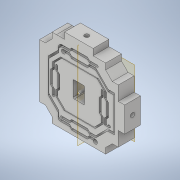
# Autodesk Inventor part: 20_Cube_Inser_Flexuremanipulator_m3_lc_fibermount_v3
Saved by Autodesk Inventor 2022 (Build 260153000, 153)
## iProperties
Created: 2021-03-01
Part Number: 20_Cube_Inser_Flexuremanipulator_m3_lc_fibermount_v3
Material: Generic
Document SubType Name: Modeling
Designer: diederichbenedict
Density: 1 g/cm^3
Appearance: Default
Author: diederichbenedict
Autodesk Inventor part; units mm, degrees
ref_plane "YZ Plane" through (0, 0, 0) normal (1, 0, 0) x (0, 1, 0)
ref_plane "XZ Plane" through (0, 0, 0) normal (0, 1, 0) x (-1, 0, 0)
ref_plane "XY Plane" through (0, 0, 0) normal (0, 0, 1) x (1, 0, 0)
ref_plane "Work Plane1" through (7.88, 34.1, 0) normal (0, 0, 1) x (-1, 0, 0)
sketch "Sketch1" plane through (7.88, 34.1, 0) normal (0, 0, 1) x (-1, 0, 0)
  circle A0 centre (24.85, 16.97) radius 1.6106 projected
  line L0 (10.689, 37.795) -> (10.689, 41.96) projected
  line L1 (10.689, 37.795) -> (10.689, 34.7795) projected
  line L2 (10.689, 34.7795) -> (7.0405, 31.131) projected
  line L3 (7.0405, 31.131) -> (4.025, 31.131) projected
  line L4 (4.025, 31.131) -> (-0.14, 31.131) projected
  line L5 (-0.14, 31.131) -> (-0.14, 2.809) projected
  line L6 (-0.14, 2.809) -> (4.025, 2.809) projected
  line L7 (4.025, 2.809) -> (7.0405, 2.809) projected
  line L8 (7.0405, 2.809) -> (10.689, -0.8395) projected
  line L9 (10.689, -0.8395) -> (10.689, -3.855) projected
  line L10 (10.689, -3.855) -> (10.689, -8.02) projected
  line L11 (10.689, -8.02) -> (39.011, -8.02) projected
  line L12 (39.011, -8.02) -> (39.011, -3.855) projected
  line L13 (39.011, -3.855) -> (39.011, -0.8395) projected
  line L14 (39.011, -0.8395) -> (42.6595, 2.809) projected
  line L15 (42.6595, 2.809) -> (45.675, 2.809) projected
  line L16 (45.675, 2.809) -> (45.675, 31.131) projected
  line L17 (42.6595, 31.131) -> (45.675, 31.131) projected
  line L18 (42.6595, 31.131) -> (39.011, 34.7795) projected
  line L19 (39.011, 34.7795) -> (39.011, 37.795) projected
  line L20 (39.011, 41.96) -> (39.011, 37.795) projected
  line L21 (10.689, 41.96) -> (39.011, 41.96) projected
  line L22 (30.605, 38.2115) -> (36.5749, 38.2115) projected
  arc A1 (37.9461, 36.6239) -> (36.5749, 38.2115) centre (36.5749, 36.8256) ccw projected
  line L23 (37.9461, 36.6239) -> (37.9461, 33.9428) projected
  line L24 (44.1756, 27.7133) -> (37.9461, 33.9428) projected
  line L25 (44.1756, 6.1367) -> (44.1756, 27.7133) projected
  line L26 (37.9461, -0.0928) -> (44.1756, 6.1367) projected
  line L27 (37.9461, -0.0928) -> (37.9461, -1.4371) projected
  arc A2 (36.0225, -4.2715) -> (37.9461, -1.4371) centre (34.8961, -1.4371) ccw projected
  line L28 (36.0225, -4.2715) -> (30.605, -4.2715) projected
  line L29 (29.3555, -5.521) -> (30.605, -4.2715) projected
  line L30 (19.3595, -5.521) -> (29.3555, -5.521) projected
  line L31 (18.11, -4.2715) -> (19.3595, -5.521) projected
  line L32 (13.2194, -4.2715) -> (18.11, -4.2715) projected
  arc A3 (13.2194, -3.022) -> (13.2194, -4.2715) centre (13.2194, -3.6467) ccw projected
  line L33 (18.11, -3.022) -> (13.2194, -3.022) projected
  line L34 (19.3595, -4.2715) -> (18.11, -3.022) projected
  line L35 (29.3555, -4.2715) -> (19.3595, -4.2715) projected
  line L36 (30.605, -3.022) -> (29.3555, -4.2715) projected
  line L37 (30.605, -3.022) -> (34.8506, -3.022) projected
  arc A4 (34.8506, -3.022) -> (37.5296, -0.9944) centre (34.8506, -0.2385) ccw projected
  line L38 (37.5296, -0.9944) -> (37.5296, 1.1567) projected
  line L39 (43.7591, 7.3862) -> (37.5296, 1.1567) projected
  line L40 (43.7591, 26.4638) -> (43.7591, 7.3862) projected
  line L41 (37.5296, 32.6933) -> (43.7591, 26.4638) projected
  line L42 (37.5296, 35.8344) -> (37.5296, 32.6933) projected
  arc A5 (37.5296, 35.8344) -> (36.402, 36.962) centre (36.402, 35.8344) ccw projected
  line L43 (30.605, 36.962) -> (36.402, 36.962) projected
  line L44 (29.3555, 38.2115) -> (30.605, 36.962) projected
  line L45 (19.3595, 38.2115) -> (29.3555, 38.2115) projected
  line L46 (18.11, 36.962) -> (19.3595, 38.2115) projected
  line L47 (14.4288, 36.962) -> (18.11, 36.962) projected
  arc A6 (15.7715, 38.3046) -> (14.4288, 36.962) centre (14.4288, 38.3046) ccw projected
  line L48 (15.7715, 38.2115) -> (15.7715, 38.3046) projected
  line L49 (18.11, 38.2115) -> (15.7715, 38.2115) projected
  line L50 (19.3595, 39.461) -> (18.11, 38.2115) projected
  line L51 (29.3555, 39.461) -> (19.3595, 39.461) projected
  line L52 (30.605, 38.2115) -> (29.3555, 39.461) projected
  line L53 (6.524, 28.5756) -> (14.0774, 36.129) projected
  line L54 (14.0774, 36.129) -> (18.11, 36.129) projected
  line L55 (18.11, 36.129) -> (19.3595, 34.8795) projected
  line L56 (19.3595, 34.8795) -> (29.3555, 34.8795) projected
  line L57 (29.3555, 34.8795) -> (30.605, 36.129) projected
  line L58 (30.605, 36.129) -> (35.7862, 36.129) projected
  arc A7 (35.7862, 34.8795) -> (35.7862, 36.129) centre (35.7862, 35.5043) ccw projected
  line L59 (35.7862, 34.8795) -> (30.605, 34.8795) projected
  line L60 (30.605, 34.8795) -> (29.3555, 33.63) projected
  line L61 (29.3555, 33.63) -> (19.3595, 33.63) projected
  line L62 (19.3595, 33.63) -> (18.11, 34.8795) projected
  line L63 (18.11, 34.8795) -> (14.0774, 34.8795) projected
  line L64 (14.0774, 34.8795) -> (6.524, 27.3261) projected
  line L65 (6.524, 27.3261) -> (2.7755, 27.3261) projected
  line L66 (2.7755, 27.3261) -> (2.7755, 6.9149) projected
  line L67 (2.7755, 6.9149) -> (6.223, 6.9149) projected
  line L68 (6.223, 6.9149) -> (14.0774, -0.9395) projected
  line L69 (14.0774, -0.9395) -> (18.11, -0.9395) projected
  line L70 (18.11, -0.9395) -> (19.3595, 0.31) projected
  line L71 (19.3595, 0.31) -> (29.3555, 0.31) projected
  line L72 (29.3555, 0.31) -> (30.605, -0.9395) projected
  line L73 (30.605, -0.9395) -> (33.3749, -0.9395) projected
  arc A8 (34.6244, -2.189) -> (33.3749, -0.9395) centre (34.6244, -0.9395) ccw projected
  line L74 (34.6244, -2.189) -> (30.605, -2.189) projected
  line L75 (30.605, -2.189) -> (29.3555, -0.9395) projected
  line L76 (29.3555, -0.9395) -> (19.3595, -0.9395) projected
  line L77 (19.3595, -0.9395) -> (18.11, -2.189) projected
  line L78 (18.11, -2.189) -> (14.0774, -2.189) projected
  line L79 (14.0774, -2.189) -> (6.223, 5.6654) projected
  line L80 (2.359, 5.6654) -> (6.223, 5.6654) projected
  line L81 (2.359, 28.5756) -> (2.359, 5.6654) projected
  line L82 (6.524, 28.5756) -> (2.359, 28.5756) projected
  line L83 (7.357, 21.135) -> (7.357, 12.805) projected
  line L84 (8.6065, 11.5555) -> (7.357, 12.805) projected
  line L85 (8.6065, 9.1359) -> (8.6065, 11.5555) projected
  line L86 (8.6065, 7.7897) -> (8.6065, 9.1359) projected
  line L87 (13.1707, 3.2255) -> (8.6065, 7.7897) projected
  line L88 (35.5512, 3.2255) -> (13.1707, 3.2255) projected
  line L89 (40.2764, 7.9507) -> (35.5512, 3.2255) projected
  line L90 (40.2764, 11.5555) -> (40.2764, 7.9507) projected
  line L91 (41.5259, 12.805) -> (40.2764, 11.5555) projected
  line L92 (41.5259, 21.135) -> (41.5259, 12.805) projected
  line L93 (40.2764, 22.3845) -> (41.5259, 21.135) projected
  line L94 (40.2764, 26.4297) -> (40.2764, 22.3845) projected
  arc A9 (41.5259, 26.4297) -> (40.2764, 26.4297) centre (40.9011, 26.4297) ccw projected
  line L95 (41.5259, 22.3845) -> (41.5259, 26.4297) projected
  line L96 (42.7754, 21.135) -> (41.5259, 22.3845) projected
  line L97 (42.7754, 12.805) -> (42.7754, 21.135) projected
  line L98 (41.5259, 11.5555) -> (42.7754, 12.805) projected
  line L99 (41.5259, 8.0241) -> (41.5259, 11.5555) projected
  line L100 (36.3107, 2.809) -> (41.5259, 8.0241) projected
  line L101 (12.3377, 2.809) -> (36.3107, 2.809) projected
  line L102 (7.357, 7.7897) -> (12.3377, 2.809) projected
  line L103 (7.357, 9.1113) -> (7.357, 7.7897) projected
  line L104 (7.357, 11.5555) -> (7.357, 9.1113) projected
  line L105 (6.1075, 12.805) -> (7.357, 11.5555) projected
  line L106 (6.1075, 21.135) -> (6.1075, 12.805) projected
  line L107 (7.357, 22.3845) -> (6.1075, 21.135) projected
  line L108 (7.357, 25.5514) -> (7.357, 22.3845) projected
  line L109 (6.3945, 25.5514) -> (7.357, 25.5514) projected
  arc A10 (5.61, 26.3074) -> (6.3945, 25.5514) centre (5.61, 25.5223) ccw projected
  line L110 (8.6065, 26.3074) -> (5.61, 26.3074) projected
  line L111 (8.6065, 22.3845) -> (8.6065, 26.3074) projected
  line L112 (7.357, 21.135) -> (8.6065, 22.3845) projected
  line L113 (9.4395, 8.2659) -> (9.4395, 11.5555) projected
  line L114 (9.4395, 11.5555) -> (10.689, 12.805) projected
  line L115 (10.689, 12.805) -> (10.689, 21.135) projected
  line L116 (10.689, 21.135) -> (9.4395, 22.3845) projected
  line L117 (9.4395, 22.3845) -> (9.4395, 26.2659) projected
  line L118 (9.4395, 26.2659) -> (14.3046, 31.131) projected
  line L119 (14.3046, 31.131) -> (34.1168, 31.131) projected
  line L120 (34.1168, 31.131) -> (39.4434, 25.8045) projected
  line L121 (39.4434, 25.8045) -> (39.4434, 22.3845) projected
  line L122 (39.4434, 22.3845) -> (38.1939, 21.135) projected
  line L123 (38.1939, 21.135) -> (38.1939, 12.805) projected
  line L124 (38.1939, 12.805) -> (39.4434, 11.5555) projected
  line L125 (39.4434, 11.5555) -> (39.4434, 8.8128) projected
  arc A11 (38.1939, 8.8128) -> (39.4434, 8.8128) centre (38.8186, 8.8128) ccw projected
  line L126 (38.1939, 8.8128) -> (38.1939, 11.5555) projected
  line L127 (38.1939, 11.5555) -> (36.9444, 12.805) projected
  line L128 (36.9444, 12.805) -> (36.9444, 21.135) projected
  line L129 (36.9444, 21.135) -> (38.1939, 22.3845) projected
  line L130 (38.1939, 22.3845) -> (38.1939, 25.8045) projected
  line L131 (38.1939, 25.8045) -> (33.2838, 30.7145) projected
  line L132 (33.2838, 30.7145) -> (15.1376, 30.7145) projected
  line L133 (15.1376, 30.7145) -> (10.689, 26.2659) projected
  line L134 (10.689, 26.2659) -> (10.689, 22.3845) projected
  line L135 (10.689, 22.3845) -> (11.9385, 21.135) projected
  line L136 (11.9385, 21.135) -> (11.9385, 12.805) projected
  line L137 (11.9385, 12.805) -> (10.689, 11.5555) projected
  line L138 (10.689, 11.5555) -> (10.689, 8.2659) projected
  arc A12 (9.4395, 8.2659) -> (10.689, 8.2659) centre (10.0643, 8.2659) ccw projected
  line L139 (7.88, -4.18) -> (3.7, 0) construction
  line L140 (7.88, 38.28) -> (3.7, 34.1) projected
  line L141 (46, 34.1) -> (41.82, 38.28) construction
  line L142 (46, 0) -> (41.82, -4.18) construction
  line L143 (41.82, -8) -> (41.82, -4.18) construction
  line L144 (46, 0) -> (49.7, 0) construction
  line L145 (46, 34.1) -> (49.7, 34.1) construction
  line L146 (41.82, 42.1) -> (41.82, 38.28) construction
  line L147 (7.88, 42.1) -> (7.88, 38.28) construction
  line L148 (0, 34.1) -> (4.1, 34.1) construction
  line L149 (3.7, 0) -> (0, 0) construction
  line L150 (7.88, -8) -> (7.88, -4.18) construction
  line L151 (39.011, -8.02) -> (41.82, -8)
  line L152 (41.82, -8) -> (41.793, -4.207)
  line L153 (46, 0) -> (41.793, -4.207)
  line L154 (10.689, -8.02) -> (7.88, -8.02)
  line L155 (7.88, -8.02) -> (7.88, -4.207)
  line L156 (7.88, -4.207) -> (3.7, 0)
  line L157 (3.7, 0) -> (0, 0)
  line L158 (0, 0) -> (-0.14, 0)
  line L159 (-0.14, 0) -> (-0.14, 2.809)
  line L160 (-0.14, 31.131) -> (-0.14, 34.1)
  line L161 (-0.14, 34.1) -> (3.7, 34.1)
  line L162 (7.88, 38.28) -> (7.88, 41.96)
  line L163 (7.88, 38.28) -> (11.56, 38.28) construction
  line L164 (7.88, 41.96) -> (10.689, 41.96)
  line L165 (39.011, 41.96) -> (41.82, 41.96)
  line L166 (41.82, 41.96) -> (41.82, 38.28)
  line L167 (46, 34.1) -> (41.82, 38.28)
  line L168 (46, 34.1) -> (49.7, 34.1)
  line L169 (49.7, 34.1) -> (49.7, 0)
  line L170 (49.7, 0) -> (46, 0)
  point P0 (7.88, 34.1)
  dimension "d0" = 0
  dimension "d1" = 90
  constraints: 40 end point, 7 perpendicular, 6 point on line, 3 collinear, 1 horizontal, 1 vertical
  measures "d0" distance from line of L154.end L150
  measures "d1" angle of L163 L162
extrude "Extrusion1" add sketch "Sketch1" along normal blind 10
sketch "Sketch3" plane through (8.02, 0, 0) normal (1, 0, 0) x (0, 0, -1)
  line L0 (0, 0) -> (0, 34.1) projected
  line L1 (0, 34.1) -> (-10, 34.1) projected
  line L2 (-10, 0) -> (-10, 34.1) projected
  line L3 (0, 0) -> (-10, 0) projected
  line L4 (0, 21.295) -> (0, 12.965) projected
  line L5 (0, 21.295) -> (-10, 21.295) projected
  line L6 (-10, 12.965) -> (-10, 21.295) projected
  line L7 (0, 12.965) -> (-10, 12.965) projected
  point P0 (0, 0)
  point P1 (-5, 17.13)
hole "Hole1" at (8.02, 17.13, 5) direction (-1, 0, 0) diameter 4.9 depth 12.0785
sketch "Sketch6" plane through (5.1045, 6.7739, 0) normal (1, 0, 0) x (0, 0, -1)
  line L0 (0, 14.5211) -> (0, 6.1911) projected
  line L1 (0, 14.5211) -> (-10, 14.5211) projected
  line L2 (-10, 6.1911) -> (-10, 14.5211) projected
  line L3 (0, 6.1911) -> (-10, 6.1911) projected
  circle A0 centre (-5, 10.3561) radius 2.45 projected
  line L4 (-5, 8.8561) -> (-5, 11.8561) construction
  line L5 (-2.2, 8.8561) -> (-2.2, 11.8561)
  line L6 (-7.8, 11.8561) -> (-7.8, 8.8561)
  arc A1 (-7.8, 8.8561) -> (-2.2, 8.8561) centre (-5, 8.8561) ccw
  arc A2 (-2.2, 11.8561) -> (-7.8, 11.8561) centre (-5, 11.8561) ccw
  line L7 (-5, 10.3561) -> (-2, 10.3561) construction
  point P0 (0, -6.7739)
  dimension "d21" = 1.5
  dimension "d22" = 90
  dimension "d23" = 5.6
  constraints: 10 end point, 4 point on circle, 4 tangent, 2 centre point, 1 horizontal, 1 midpoint, 1 parallel, 1 perpendicular, 1 vertical
  measures "d21" distance of L7.start L4.end
  measures "d22" angle of L7 L4
  measures "d23" diameter of A2
extrude "Extrusion4" cut sketch "Sketch6" against normal up to surface (7.9135 mm away) contours A2 L5 A1 L3 L6 L1 | L1 A2 | A1 L3 | A0
pattern_circular "Circular Pattern3" count 2 over 90 about axis through (-16.97, 17.13, 0) along (0, 0, 1) of "Hole1", "Extrusion4"
sketch "Sketch7" plane through (7.88, 34.1, 10) normal (0, 0, 1) x (1, 0, 0)
  arc A0 (-37.9461, -36.6239) -> (-36.5749, -38.2115) centre (-36.5749, -36.8256) ccw projected
  line L0 (-37.9461, -36.6239) -> (-37.9461, -33.9428) projected
  line L1 (-37.9461, -33.9428) -> (-44.1756, -27.7133) projected
  line L2 (-44.1756, -27.7133) -> (-44.1756, -6.1367) projected
  line L3 (-44.1756, -6.1367) -> (-37.9461, 0.0928) projected
  line L4 (-37.9461, 0.0928) -> (-37.9461, 1.4371) projected
  arc A1 (-36.0225, 4.2715) -> (-37.9461, 1.4371) centre (-34.8961, 1.4371) ccw projected
  line L5 (-36.0225, 4.2715) -> (-30.605, 4.2715) projected
  line L6 (-30.605, 4.2715) -> (-29.3555, 5.521) projected
  line L7 (-29.3555, 5.521) -> (-19.3595, 5.521) projected
  line L8 (-19.3595, 5.521) -> (-18.11, 4.2715) projected
  line L9 (-18.11, 4.2715) -> (-13.2194, 4.2715) projected
  arc A2 (-13.2194, 3.022) -> (-13.2194, 4.2715) centre (-13.2194, 3.6467) ccw projected
  line L10 (-13.2194, 3.022) -> (-18.11, 3.022) projected
  line L11 (-18.11, 3.022) -> (-19.3595, 4.2715) projected
  line L12 (-19.3595, 4.2715) -> (-29.3555, 4.2715) projected
  line L13 (-29.3555, 4.2715) -> (-30.605, 3.022) projected
  line L14 (-30.605, 3.022) -> (-34.8506, 3.022) projected
  arc A3 (-34.8506, 3.022) -> (-37.5296, 0.9944) centre (-34.8506, 0.2385) ccw projected
  line L15 (-37.5296, 0.9944) -> (-37.5296, -1.1567) projected
  line L16 (-37.5296, -1.1567) -> (-43.7591, -7.3862) projected
  line L17 (-43.7591, -7.3862) -> (-43.7591, -26.4638) projected
  line L18 (-43.7591, -26.4638) -> (-37.5296, -32.6933) projected
  line L19 (-37.5296, -32.6933) -> (-37.5296, -35.8344) projected
  arc A4 (-37.5296, -35.8344) -> (-36.402, -36.962) centre (-36.402, -35.8344) ccw projected
  line L20 (-36.402, -36.962) -> (-30.605, -36.962) projected
  line L21 (-30.605, -36.962) -> (-29.3555, -38.2115) projected
  line L22 (-29.3555, -38.2115) -> (-19.3595, -38.2115) projected
  line L23 (-19.3595, -38.2115) -> (-18.11, -36.962) projected
  line L24 (-18.11, -36.962) -> (-14.4288, -36.962) projected
  arc A5 (-15.7715, -38.3046) -> (-14.4288, -36.962) centre (-14.4288, -38.3046) ccw projected
  line L25 (-15.7715, -38.3046) -> (-15.7715, -38.2115) projected
  line L26 (-15.7715, -38.2115) -> (-18.11, -38.2115) projected
  line L27 (-18.11, -38.2115) -> (-19.3595, -39.461) projected
  line L28 (-19.3595, -39.461) -> (-29.3555, -39.461) projected
  line L29 (-29.3555, -39.461) -> (-30.605, -38.2115) projected
  line L30 (-30.605, -38.2115) -> (-36.5749, -38.2115) projected
  line L31 (-14.0774, -36.129) -> (-18.11, -36.129) projected
  line L32 (-18.11, -36.129) -> (-19.3595, -34.8795) projected
  line L33 (-19.3595, -34.8795) -> (-29.3555, -34.8795) projected
  line L34 (-29.3555, -34.8795) -> (-30.605, -36.129) projected
  line L35 (-30.605, -36.129) -> (-35.7862, -36.129) projected
  arc A6 (-35.7862, -34.8795) -> (-35.7862, -36.129) centre (-35.7862, -35.5043) ccw projected
  line L36 (-35.7862, -34.8795) -> (-30.605, -34.8795) projected
  line L37 (-30.605, -34.8795) -> (-29.3555, -33.63) projected
  line L38 (-29.3555, -33.63) -> (-19.3595, -33.63) projected
  line L39 (-19.3595, -33.63) -> (-18.11, -34.8795) projected
  line L40 (-18.11, -34.8795) -> (-14.0774, -34.8795) projected
  line L41 (-14.0774, -34.8795) -> (-6.524, -27.3261) projected
  line L42 (-6.524, -27.3261) -> (-2.7755, -27.3261) projected
  line L43 (-2.7755, -27.3261) -> (-2.7755, -6.9149) projected
  line L44 (-2.7755, -6.9149) -> (-6.223, -6.9149) projected
  line L45 (-6.223, -6.9149) -> (-14.0774, 0.9395) projected
  line L46 (-14.0774, 0.9395) -> (-18.11, 0.9395) projected
  line L47 (-18.11, 0.9395) -> (-19.3595, -0.31) projected
  line L48 (-19.3595, -0.31) -> (-29.3555, -0.31) projected
  line L49 (-29.3555, -0.31) -> (-30.605, 0.9395) projected
  line L50 (-30.605, 0.9395) -> (-33.3749, 0.9395) projected
  arc A7 (-34.6244, 2.189) -> (-33.3749, 0.9395) centre (-34.6244, 0.9395) ccw projected
  line L51 (-34.6244, 2.189) -> (-30.605, 2.189) projected
  line L52 (-30.605, 2.189) -> (-29.3555, 0.9395) projected
  line L53 (-29.3555, 0.9395) -> (-19.3595, 0.9395) projected
  line L54 (-19.3595, 0.9395) -> (-18.11, 2.189) projected
  line L55 (-18.11, 2.189) -> (-14.0774, 2.189) projected
  line L56 (-14.0774, 2.189) -> (-6.223, -5.6654) projected
  line L57 (-6.223, -5.6654) -> (-2.359, -5.6654) projected
  line L58 (-2.359, -5.6654) -> (-2.359, -28.5756) projected
  line L59 (-2.359, -28.5756) -> (-6.524, -28.5756) projected
  line L60 (-6.524, -28.5756) -> (-14.0774, -36.129) projected
  line L61 (-7.357, -12.805) -> (-8.6065, -11.5555) projected
  line L62 (-8.6065, -11.5555) -> (-8.6065, -7.7897) projected
  line L63 (-8.6065, -7.7897) -> (-13.1707, -3.2255) projected
  line L64 (-13.1707, -3.2255) -> (-35.5512, -3.2255) projected
  line L65 (-35.5512, -3.2255) -> (-40.2764, -7.9507) projected
  line L66 (-40.2764, -7.9507) -> (-40.2764, -11.5555) projected
  line L67 (-40.2764, -11.5555) -> (-41.5259, -12.805) projected
  line L68 (-41.5259, -12.805) -> (-41.5259, -21.135) projected
  line L69 (-41.5259, -21.135) -> (-40.2764, -22.3845) projected
  line L70 (-40.2764, -22.3845) -> (-40.2764, -26.4297) projected
  arc A8 (-41.5259, -26.4297) -> (-40.2764, -26.4297) centre (-40.9011, -26.4297) ccw projected
  line L71 (-41.5259, -26.4297) -> (-41.5259, -22.3845) projected
  line L72 (-41.5259, -22.3845) -> (-42.7754, -21.135) projected
  line L73 (-42.7754, -21.135) -> (-42.7754, -12.805) projected
  line L74 (-42.7754, -12.805) -> (-41.5259, -11.5555) projected
  line L75 (-41.5259, -11.5555) -> (-41.5259, -8.0241) projected
  line L76 (-41.5259, -8.0241) -> (-36.3107, -2.809) projected
  line L77 (-36.3107, -2.809) -> (-12.3377, -2.809) projected
  line L78 (-12.3377, -2.809) -> (-7.357, -7.7897) projected
  line L79 (-7.357, -7.7897) -> (-7.357, -11.5555) projected
  line L80 (-7.357, -11.5555) -> (-6.1075, -12.805) projected
  line L81 (-6.1075, -12.805) -> (-6.1075, -21.135) projected
  line L82 (-6.1075, -21.135) -> (-7.357, -22.3845) projected
  line L83 (-7.357, -22.3845) -> (-7.357, -25.5514) projected
  line L84 (-7.357, -25.5514) -> (-6.3945, -25.5514) projected
  arc A9 (-5.61, -26.3074) -> (-6.3945, -25.5514) centre (-5.61, -25.5223) ccw projected
  line L85 (-5.61, -26.3074) -> (-8.6065, -26.3074) projected
  line L86 (-8.6065, -26.3074) -> (-8.6065, -22.3845) projected
  line L87 (-8.6065, -22.3845) -> (-7.357, -21.135) projected
  line L88 (-7.357, -21.135) -> (-7.357, -12.805) projected
  line L89 (-9.4395, -11.5555) -> (-10.689, -12.805) projected
  line L90 (-10.689, -12.805) -> (-10.689, -21.135) projected
  line L91 (-10.689, -21.135) -> (-9.4395, -22.3845) projected
  line L92 (-9.4395, -22.3845) -> (-9.4395, -26.2659) projected
  line L93 (-9.4395, -26.2659) -> (-14.3046, -31.131) projected
  line L94 (-14.3046, -31.131) -> (-34.1168, -31.131) projected
  line L95 (-34.1168, -31.131) -> (-39.4434, -25.8045) projected
  line L96 (-39.4434, -25.8045) -> (-39.4434, -22.3845) projected
  line L97 (-39.4434, -22.3845) -> (-38.1939, -21.135) projected
  line L98 (-38.1939, -21.135) -> (-38.1939, -12.805) projected
  line L99 (-38.1939, -12.805) -> (-39.4434, -11.5555) projected
  line L100 (-39.4434, -11.5555) -> (-39.4434, -8.8128) projected
  arc A10 (-38.1939, -8.8128) -> (-39.4434, -8.8128) centre (-38.8186, -8.8128) ccw projected
  line L101 (-38.1939, -8.8128) -> (-38.1939, -11.5555) projected
  line L102 (-38.1939, -11.5555) -> (-36.9444, -12.805) projected
  line L103 (-36.9444, -12.805) -> (-36.9444, -21.135) projected
  line L104 (-36.9444, -21.135) -> (-38.1939, -22.3845) projected
  line L105 (-38.1939, -22.3845) -> (-38.1939, -25.8045) projected
  line L106 (-38.1939, -25.8045) -> (-33.2838, -30.7145) projected
  line L107 (-33.2838, -30.7145) -> (-15.1376, -30.7145) projected
  line L108 (-15.1376, -30.7145) -> (-10.689, -26.2659) projected
  line L109 (-10.689, -26.2659) -> (-10.689, -22.3845) projected
  line L110 (-10.689, -22.3845) -> (-11.9385, -21.135) projected
  line L111 (-11.9385, -21.135) -> (-11.9385, -12.805) projected
  line L112 (-11.9385, -12.805) -> (-10.689, -11.5555) projected
  line L113 (-10.689, -11.5555) -> (-10.689, -8.2659) projected
  arc A11 (-9.4395, -8.2659) -> (-10.689, -8.2659) centre (-10.0643, -8.2659) ccw projected
  line L114 (-9.4395, -8.2659) -> (-9.4395, -11.5555) projected
  circle A12 centre (-24.85, -16.97) radius 1.6106 projected
  line L115 (-41.82, -41.96) -> (-7.88, -41.96) projected
  line L116 (-7.88, -41.96) -> (-7.88, -38.28) projected
  line L117 (-7.88, -38.28) -> (-3.7, -34.1) projected
  line L118 (-3.7, -34.1) -> (0.14, -34.1) projected
  line L119 (0.14, -34.1) -> (0.14, 0) projected
  line L120 (0.14, 0) -> (-3.7, 0) projected
  line L121 (-3.7, 0) -> (-7.88, 4.207) projected
  line L122 (-7.88, 4.207) -> (-7.88, 8.02) projected
  line L123 (-7.88, 8.02) -> (-39.011, 8.02) projected
  line L124 (-39.011, 8.02) -> (-41.82, 8) projected
  line L125 (-41.82, 8) -> (-41.793, 4.207) projected
  line L126 (-41.793, 4.207) -> (-46, 0) projected
  line L127 (-46, 0) -> (-49.7, 0) projected
  line L128 (-49.7, 0) -> (-49.7, -34.1) projected
  line L129 (-49.7, -34.1) -> (-46, -34.1) projected
  line L130 (-46, -34.1) -> (-41.82, -38.28) projected
  line L131 (-41.82, -38.28) -> (-41.82, -41.96) projected
  circle A13 centre (-24.85, -16.97) radius 9.75
  point P0 (-7.88, -34.1)
  dimension "d32" = 19.5
  dimension "d33" = 0
  dimension "d34" = 0
  constraints: 1 centre point
  measures "d32" diameter of A13
  measures "d33" distance of A13.centre A12.centre
  measures "d34" distance of A12.centre A13.centre
extrude "Extrusion5" cut sketch "Sketch7" against normal through all contours A13
ref_plane "Work Plane2" through (-16.97, 17.13, 10) normal (1, 0, 0) x (0, 0, -1)
sketch "Sketch8" plane through (-16.97, 17.13, 10) normal (1, 0, 0) x (0, 0, -1)
  line L0 (15.6463, -9.95) -> (15.7963, -9.95)
  line L1 (15.6463, -9.95) -> (15.7963, -9.95) construction
  line L2 (15.7963, -9.95) -> (16.003, -10.308)
  line L3 (16.003, -10.308) -> (16.153, -10.308)
  line L4 (16.153, -10.308) -> (16.3596, -9.95)
  line L5 (16.3596, -9.95) -> (16.3596, -10.95)
  line L6 (16.3596, -10.95) -> (15.6463, -10.95)
  line L7 (15.6463, -10.95) -> (15.6463, -9.95)
  line L8 (0, -9.75) -> (10, -9.75) projected
  line L9 (15.6463, -9.95) -> (15.6463, -8.6204)
  line L10 (15.6463, -8.6204) -> (16.3596, -8.6204)
  line L11 (16.3596, -8.6204) -> (16.3596, -9.95)
  line L12 (-0.4283, 0) -> (15.6742, 0)
  point P0 (10, -17.13)
  dimension "d37" = 0.15
  dimension "d38" = 0
  dimension "d39" = 120
  dimension "d40" = 0.15
  dimension "d41" = 120
  dimension "d42" = 1
  dimension "d43" = 0.7133
  dimension "d44" = 9.95
  dimension "d45" = 9.75
  constraints: 24 end point, 3 horizontal, 3 perpendicular, 2 parallel, 1 collinear, 1 point on line
  measures "d37" distance of L0.start L0.end
  measures "d38" distance between parallel lines of L0 L1
  measures "d39" angle of L0 L2
  measures "d40" distance of L2.end L3.end
  measures "d41" angle of L4 L3
  measures "d42" distance of L4.end L5.end
  measures "d43" distance between parallel lines of L7 L5
  measures "d44" distance from line of L12.end L0
  measures "d45" distance from line of L12.end L8
coil "Coil1" sketch "Sketch8" operation cut axis through (-16.97, 17.13, 10.4283) along (0, 0, 1) pitch 0.7133 turns 30 hand right contours L9 L10 L11 L4 L3 L2 L0
sketch "Sketch9" plane through (8.02, 0, 0) normal (1, 0, 0) x (0, 0, -1)
  circle A0 centre (-5, 17.13) radius 2.45 projected
  line L0 (-10, 25.13) -> (0, 25.13)
  line L1 (0, 25.13) -> (0, 9.13)
  line L2 (0, 9.13) -> (-10, 9.13)
  line L3 (-10, 9.13) -> (-10, 25.13)
  line L4 (-10, 25.13) -> (0, 9.13) construction
  line L5 (0, 25.13) -> (-10, 9.13) construction
  point P0 (0, 0)
  dimension "d55" = 10
  dimension "d56" = 16
  constraints: 12 end point, 2 midpoint, 2 parallel, 1 horizontal, 1 perpendicular
  measures "d55" distance of L1.end L2.end
  measures "d56" distance of L0.end L1.end
extrude "Extrusion6" add sketch "Sketch9" along normal blind 4
sketch "Sketch10" plane through (-31.131, 42.12, 0) normal (0, 1, 0) x (1, 0, 0)
  circle A0 centre (14.161, -5) radius 2.45 projected
  line L0 (5.161, 0) -> (23.161, 0)
  line L1 (23.161, 0) -> (23.161, -10)
  line L2 (23.161, -10) -> (5.161, -10)
  line L3 (5.161, -10) -> (5.161, 0)
  line L4 (5.161, 0) -> (23.161, -10) construction
  line L5 (23.161, 0) -> (5.161, -10) construction
  point P0 (31.131, 0)
  dimension "d59" = 18
  dimension "d60" = 10
  constraints: 12 end point, 2 midpoint, 2 parallel, 1 horizontal, 1 perpendicular
  measures "d59" distance of L1.end L2.end
  measures "d60" distance of L0.end L1.end
extrude "Extrusion7" add sketch "Sketch10" along normal blind 4
sketch "Sketch12" plane through (7.88, 34.1, 0) normal (0, 0, -1) x (-1, 0, 0)
  arc A0 (17.7858, -23.9771) -> (29.8952, -25.546) centre (24.85, -16.97) ccw projected
  arc A1 (32.1684, -9.7109) -> (19.6233, -8.0855) centre (24.85, -16.97) ccw projected
  arc A2 (36.5749, -38.2115) -> (37.9461, -36.6239) centre (36.5749, -36.8256) ccw projected
  line L0 (36.5749, -38.2115) -> (30.605, -38.2115) projected
  line L1 (30.605, -38.2115) -> (29.3555, -39.461) projected
  line L2 (29.3555, -39.461) -> (19.3595, -39.461) projected
  line L3 (19.3595, -39.461) -> (18.11, -38.2115) projected
  line L4 (18.11, -38.2115) -> (15.7715, -38.2115) projected
  line L5 (15.7715, -38.2115) -> (15.7715, -38.3046) projected
  arc A3 (14.4288, -36.962) -> (15.7715, -38.3046) centre (14.4288, -38.3046) ccw projected
  line L6 (14.4288, -36.962) -> (18.11, -36.962) projected
  line L7 (18.11, -36.962) -> (19.3595, -38.2115) projected
  line L8 (19.3595, -38.2115) -> (29.3555, -38.2115) projected
  line L9 (29.3555, -38.2115) -> (30.605, -36.962) projected
  line L10 (30.605, -36.962) -> (36.402, -36.962) projected
  arc A4 (36.402, -36.962) -> (37.5296, -35.8344) centre (36.402, -35.8344) ccw projected
  line L11 (37.5296, -35.8344) -> (37.5296, -32.6933) projected
  line L12 (37.5296, -32.6933) -> (43.7591, -26.4638) projected
  line L13 (43.7591, -26.4638) -> (43.7591, -7.3862) projected
  line L14 (43.7591, -7.3862) -> (37.5296, -1.1567) projected
  line L15 (37.5296, -1.1567) -> (37.5296, 0.9944) projected
  arc A5 (37.5296, 0.9944) -> (34.8506, 3.022) centre (34.8506, 0.2385) ccw projected
  line L16 (34.8506, 3.022) -> (30.605, 3.022) projected
  line L17 (30.605, 3.022) -> (29.3555, 4.2715) projected
  line L18 (29.3555, 4.2715) -> (19.3595, 4.2715) projected
  line L19 (19.3595, 4.2715) -> (18.11, 3.022) projected
  line L20 (18.11, 3.022) -> (13.2194, 3.022) projected
  arc A6 (13.2194, 4.2715) -> (13.2194, 3.022) centre (13.2194, 3.6467) ccw projected
  line L21 (13.2194, 4.2715) -> (18.11, 4.2715) projected
  line L22 (18.11, 4.2715) -> (19.3595, 5.521) projected
  line L23 (19.3595, 5.521) -> (29.3555, 5.521) projected
  line L24 (29.3555, 5.521) -> (30.605, 4.2715) projected
  line L25 (30.605, 4.2715) -> (36.0225, 4.2715) projected
  arc A7 (37.9461, 1.4371) -> (36.0225, 4.2715) centre (34.8961, 1.4371) ccw projected
  line L26 (37.9461, 1.4371) -> (37.9461, 0.0928) projected
  line L27 (37.9461, 0.0928) -> (44.1756, -6.1367) projected
  line L28 (44.1756, -6.1367) -> (44.1756, -27.7133) projected
  line L29 (44.1756, -27.7133) -> (37.9461, -33.9428) projected
  line L30 (37.9461, -33.9428) -> (37.9461, -36.6239) projected
  line L31 (18.11, -36.129) -> (14.0774, -36.129) projected
  line L32 (14.0774, -36.129) -> (6.524, -28.5756) projected
  line L33 (6.524, -28.5756) -> (2.359, -28.5756) projected
  line L34 (2.359, -28.5756) -> (2.359, -5.6654) projected
  line L35 (2.359, -5.6654) -> (6.223, -5.6654) projected
  line L36 (6.223, -5.6654) -> (14.0774, 2.189) projected
  line L37 (14.0774, 2.189) -> (18.11, 2.189) projected
  line L38 (18.11, 2.189) -> (19.3595, 0.9395) projected
  line L39 (19.3595, 0.9395) -> (29.3555, 0.9395) projected
  line L40 (29.3555, 0.9395) -> (30.605, 2.189) projected
  line L41 (30.605, 2.189) -> (34.6244, 2.189) projected
  arc A8 (33.3749, 0.9395) -> (34.6244, 2.189) centre (34.6244, 0.9395) ccw projected
  line L42 (33.3749, 0.9395) -> (30.605, 0.9395) projected
  line L43 (30.605, 0.9395) -> (29.3555, -0.31) projected
  line L44 (29.3555, -0.31) -> (19.3595, -0.31) projected
  line L45 (19.3595, -0.31) -> (18.11, 0.9395) projected
  line L46 (18.11, 0.9395) -> (14.0774, 0.9395) projected
  line L47 (14.0774, 0.9395) -> (6.223, -6.9149) projected
  line L48 (6.223, -6.9149) -> (2.7755, -6.9149) projected
  line L49 (2.7755, -6.9149) -> (2.7755, -27.3261) projected
  line L50 (2.7755, -27.3261) -> (6.524, -27.3261) projected
  line L51 (6.524, -27.3261) -> (14.0774, -34.8795) projected
  line L52 (14.0774, -34.8795) -> (18.11, -34.8795) projected
  line L53 (18.11, -34.8795) -> (19.3595, -33.63) projected
  line L54 (19.3595, -33.63) -> (29.3555, -33.63) projected
  line L55 (29.3555, -33.63) -> (30.605, -34.8795) projected
  line L56 (30.605, -34.8795) -> (35.7862, -34.8795) projected
  arc A9 (35.7862, -36.129) -> (35.7862, -34.8795) centre (35.7862, -35.5043) ccw projected
  line L57 (35.7862, -36.129) -> (30.605, -36.129) projected
  line L58 (30.605, -36.129) -> (29.3555, -34.8795) projected
  line L59 (29.3555, -34.8795) -> (19.3595, -34.8795) projected
  line L60 (19.3595, -34.8795) -> (18.11, -36.129) projected
  line L61 (8.6065, -11.5555) -> (7.357, -12.805) projected
  line L62 (7.357, -12.805) -> (7.357, -21.135) projected
  line L63 (7.357, -21.135) -> (8.6065, -22.3845) projected
  line L64 (8.6065, -22.3845) -> (8.6065, -26.3074) projected
  line L65 (8.6065, -26.3074) -> (5.61, -26.3074) projected
  arc A10 (6.3945, -25.5514) -> (5.61, -26.3074) centre (5.61, -25.5223) ccw projected
  line L66 (6.3945, -25.5514) -> (7.357, -25.5514) projected
  line L67 (7.357, -25.5514) -> (7.357, -22.3845) projected
  line L68 (7.357, -22.3845) -> (6.1075, -21.135) projected
  line L69 (6.1075, -21.135) -> (6.1075, -12.805) projected
  line L70 (6.1075, -12.805) -> (7.357, -11.5555) projected
  line L71 (7.357, -11.5555) -> (7.357, -7.7897) projected
  line L72 (7.357, -7.7897) -> (12.3377, -2.809) projected
  line L73 (12.3377, -2.809) -> (36.3107, -2.809) projected
  line L74 (36.3107, -2.809) -> (41.5259, -8.0241) projected
  line L75 (41.5259, -8.0241) -> (41.5259, -11.5555) projected
  line L76 (41.5259, -11.5555) -> (42.7754, -12.805) projected
  line L77 (42.7754, -12.805) -> (42.7754, -21.135) projected
  line L78 (42.7754, -21.135) -> (41.5259, -22.3845) projected
  line L79 (41.5259, -22.3845) -> (41.5259, -26.4297) projected
  arc A11 (40.2764, -26.4297) -> (41.5259, -26.4297) centre (40.9011, -26.4297) ccw projected
  line L80 (40.2764, -26.4297) -> (40.2764, -22.3845) projected
  line L81 (40.2764, -22.3845) -> (41.5259, -21.135) projected
  line L82 (41.5259, -21.135) -> (41.5259, -12.805) projected
  line L83 (41.5259, -12.805) -> (40.2764, -11.5555) projected
  line L84 (40.2764, -11.5555) -> (40.2764, -7.9507) projected
  line L85 (40.2764, -7.9507) -> (35.5512, -3.2255) projected
  line L86 (35.5512, -3.2255) -> (13.1707, -3.2255) projected
  line L87 (13.1707, -3.2255) -> (8.6065, -7.7897) projected
  line L88 (8.6065, -7.7897) -> (8.6065, -11.5555) projected
  line L89 (10.689, -12.805) -> (9.4395, -11.5555) projected
  line L90 (9.4395, -11.5555) -> (9.4395, -8.2659) projected
  arc A12 (10.689, -8.2659) -> (9.4395, -8.2659) centre (10.0643, -8.2659) ccw projected
  line L91 (10.689, -8.2659) -> (10.689, -11.5555) projected
  line L92 (10.689, -11.5555) -> (11.9385, -12.805) projected
  line L93 (11.9385, -12.805) -> (11.9385, -21.135) projected
  line L94 (11.9385, -21.135) -> (10.689, -22.3845) projected
  line L95 (10.689, -22.3845) -> (10.689, -26.2659) projected
  line L96 (10.689, -26.2659) -> (15.1376, -30.7145) projected
  line L97 (15.1376, -30.7145) -> (33.2838, -30.7145) projected
  line L98 (33.2838, -30.7145) -> (38.1939, -25.8045) projected
  line L99 (38.1939, -25.8045) -> (38.1939, -22.3845) projected
  line L100 (38.1939, -22.3845) -> (36.9444, -21.135) projected
  line L101 (36.9444, -21.135) -> (36.9444, -12.805) projected
  line L102 (36.9444, -12.805) -> (38.1939, -11.5555) projected
  line L103 (38.1939, -11.5555) -> (38.1939, -8.8128) projected
  arc A13 (39.4434, -8.8128) -> (38.1939, -8.8128) centre (38.8186, -8.8128) ccw projected
  line L104 (39.4434, -8.8128) -> (39.4434, -11.5555) projected
  line L105 (39.4434, -11.5555) -> (38.1939, -12.805) projected
  line L106 (38.1939, -12.805) -> (38.1939, -21.135) projected
  line L107 (38.1939, -21.135) -> (39.4434, -22.3845) projected
  line L108 (39.4434, -22.3845) -> (39.4434, -25.8045) projected
  line L109 (39.4434, -25.8045) -> (34.1168, -31.131) projected
  line L110 (34.1168, -31.131) -> (14.3046, -31.131) projected
  line L111 (14.3046, -31.131) -> (9.4395, -26.2659) projected
  line L112 (9.4395, -26.2659) -> (9.4395, -22.3845) projected
  line L113 (9.4395, -22.3845) -> (10.689, -21.135) projected
  line L114 (10.689, -21.135) -> (10.689, -12.805) projected
  line L115 (41.82, -41.96) -> (7.88, -41.96) projected
  line L116 (41.82, -38.28) -> (41.82, -41.96) projected
  line L117 (46, -34.1) -> (41.82, -38.28) projected
  line L118 (49.7, -34.1) -> (46, -34.1) projected
  line L119 (49.7, 0) -> (49.7, -34.1) projected
  line L120 (46, 0) -> (49.7, 0) projected
  line L121 (41.793, 4.207) -> (46, 0) projected
  line L122 (41.82, 8) -> (41.793, 4.207) projected
  line L123 (39.011, 8.02) -> (41.82, 8) projected
  line L124 (33.85, 8.02) -> (39.011, 8.02) projected
  line L125 (33.85, 8.02) -> (33.85, 12.02) projected
  line L126 (15.85, 12.02) -> (33.85, 12.02) projected
  line L127 (15.85, 8.02) -> (15.85, 12.02) projected
  line L128 (7.88, 8.02) -> (15.85, 8.02) projected
  line L129 (7.88, 4.207) -> (7.88, 8.02) projected
  line L130 (3.7, 0) -> (7.88, 4.207) projected
  line L131 (-0.14, 0) -> (3.7, 0) projected
  line L132 (-0.14, -8.97) -> (-0.14, 0) projected
  line L133 (-0.14, -8.97) -> (-4.14, -8.97) projected
  line L134 (-4.14, -24.97) -> (-4.14, -8.97) projected
  line L135 (-0.14, -24.97) -> (-4.14, -24.97) projected
  line L136 (-0.14, -34.1) -> (-0.14, -24.97) projected
  line L137 (3.7, -34.1) -> (-0.14, -34.1) projected
  line L138 (7.88, -38.28) -> (3.7, -34.1) projected
  line L139 (7.88, -41.96) -> (7.88, -38.28) projected
  circle A14 centre (24.85, -16.97) radius 0.9 projected
  line L140 (21.4, -11.87) -> (21.4, -20.97) projected
  arc A15 (21.4, -20.97) -> (21.9, -21.47) centre (21.9, -20.97) ccw projected
  line L141 (21.9, -21.47) -> (27.8, -21.47) projected
  arc A16 (27.8, -21.47) -> (28.3, -20.97) centre (27.8, -20.97) ccw projected
  line L142 (28.3, -20.97) -> (28.3, -11.87) projected
  arc A17 (28.3, -11.87) -> (27.8, -11.37) centre (27.8, -11.87) ccw projected
  line L143 (27.8, -11.37) -> (21.9, -11.37) projected
  arc A18 (21.9, -11.37) -> (21.4, -11.87) centre (21.9, -11.87) ccw projected
  line L144 (24, -19.62) -> (24, -20.17) projected
  line L145 (22.55, -19.62) -> (24, -19.62) projected
  line L146 (22.55, -15.02) -> (22.55, -19.62) projected
  line L147 (23.2, -15.02) -> (22.55, -15.02) projected
  line L148 (23.2, -14.22) -> (23.2, -15.02) projected
  line L149 (22.55, -14.22) -> (23.2, -14.22) projected
  line L150 (22.55, -13.12) -> (22.55, -14.22) projected
  line L151 (23.55, -13.12) -> (22.55, -13.12) projected
  line L152 (23.55, -12.12) -> (23.55, -13.12) projected
  line L153 (26.15, -12.12) -> (23.55, -12.12) projected
  line L154 (26.15, -13.12) -> (26.15, -12.12) projected
  line L155 (27.15, -13.12) -> (26.15, -13.12) projected
  line L156 (27.15, -14.22) -> (27.15, -13.12) projected
  line L157 (26.5, -14.22) -> (27.15, -14.22) projected
  line L158 (26.5, -15.02) -> (26.5, -14.22) projected
  line L159 (27.15, -15.02) -> (26.5, -15.02) projected
  line L160 (27.15, -19.62) -> (27.15, -15.02) projected
  line L161 (25.7, -19.62) -> (27.15, -19.62) projected
  line L162 (25.7, -20.17) -> (25.7, -19.62) projected
  line L163 (24, -20.17) -> (25.7, -20.17) projected
  line L164 (28.5, -11.87) -> (28.5, -20.97)
  arc A19 (27.8, -21.67) -> (28.5, -20.97) centre (27.8, -20.97) ccw
  line L165 (27.8, -21.67) -> (21.9, -21.67)
  arc A20 (21.2, -20.97) -> (21.9, -21.67) centre (21.9, -20.97) ccw
  line L166 (21.2, -20.97) -> (21.2, -11.87)
  arc A21 (21.9, -11.17) -> (21.2, -11.87) centre (21.9, -11.87) ccw
  line L167 (21.9, -11.17) -> (27.8, -11.17)
  arc A22 (28.5, -11.87) -> (27.8, -11.17) centre (27.8, -11.87) ccw
  circle A23 centre (24.85, -16.97) radius 10.9983
  point P0 (7.88, -34.1)
  dimension "d69" = 0.2
  constraints: 8 end point, 8 point on circle, 5 centre point, 1 coincident, 9 other
  measures "d69" distance between parallel lines of L142 L164
extrude "Extrusion9" add sketch "Sketch12" against normal up to surface (10 mm away) contours A14 | A23
sketch "Sketch13" plane through (12.02, 0, 0) normal (1, 0, 0) x (0, 0, -1)
  circle A0 centre (-5, 17.13) radius 2.45 projected
  circle A1 centre (-5, 17.13) radius 1.4
  point P0 (0, 0)
  dimension "d72" = 2.8
  constraints: 1 centre point, 1 coincident
  measures "d72" diameter of A1
extrude "Extrusion10" add sketch "Sketch13" against normal up to surface (6.499 mm away)
sketch "Sketch14" plane through (-31.131, 46.12, 0) normal (0, 1, 0) x (1, 0, 0)
  circle A0 centre (14.161, -5) radius 2.45 projected
  circle A1 centre (14.161, -5) radius 1.4
  point P0 (31.131, 0)
  dimension "d75" = 2.8
  constraints: 1 centre point, 1 coincident
  measures "d75" diameter of A1
extrude "Extrusion11" add sketch "Sketch14" against normal up to surface (6.499 mm away)
equation "\"d40\" = d37"
equation "\"d41\" = d39"
body "Solid1"
